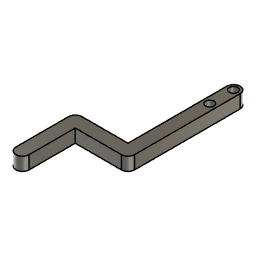
Grabing_Stick2_ver4 v4 (Autodesk Fusion 360 design; units mm, degrees)
Autodesk Fusion 360 part; units mm, degrees
sketch "스케치1" plane through (0, 0, 0) normal (0, 0, 1) x (1, 0, 0)
  line L0 (-2.5, 25) -> (-2.5, -15)
  arc A0 (-2.5, -15) -> (2.5, -15) centre (0, -15) ccw
  line L1 (2.5, -15) -> (2.5, 25)
  arc A1 (2.5, 25) -> (-2.5, 25) centre (0, 25) ccw
  line L2 (0, 25) -> (0, -15) construction
  line L3 (0, -12.5) -> (-20, -12.5)
  arc A2 (-20, -12.5) -> (-20, -17.5) centre (-20, -15) ccw
  line L4 (-20, -17.5) -> (0, -17.5)
  arc A3 (0, -17.5) -> (0, -12.5) centre (0, -15) ccw
  line L5 (0, -15) -> (-20, -15) construction
  line L6 (-22.5, -15) -> (-22.5, -35)
  arc A4 (-22.5, -35) -> (-17.5, -35) centre (-20, -35) ccw
  line L7 (-17.5, -35) -> (-17.5, -15)
  arc A5 (-17.5, -15) -> (-22.5, -15) centre (-20, -15) ccw
  line L8 (-20, -15) -> (-20, -35) construction
  circle A6 centre (0, 25) radius 1.6
  line L9 (-10, 16) -> (11, 16)
  circle A7 centre (0, 16) radius 1.6
  dimension "d1" = 5
  dimension "d2" = 5
  dimension "d3" = 5
  dimension "d4" = 3.2
  dimension "d5" = 9
  dimension "d6" = 3.2
  dimension "d9" = 20
  constraint tangent L0 A0
  constraint tangent A0 L1
  constraint parallel L0 L1
  constraint tangent L1 A1
  constraint tangent L0 A1
  constraint vertical L2
  constraint tangent L3 A2
  constraint tangent A2 L4
  constraint parallel L3 L4
  constraint tangent L4 A3
  constraint tangent L3 A3
  constraint perpendicular L2 L5
  constraint coincident A0.centre L2.end
  constraint tangent L6 A4
  constraint tangent A4 L7
  constraint parallel L6 L7
  constraint tangent L7 A5
  constraint tangent L6 A5
  constraint perpendicular L4 L8
  constraint coincident A2.centre L5.end
  constraint concentric A1 A6
  constraint perpendicular L1 L9
  constraint coincident L9 A7.centre
  constraint coincident L2 A7.centre
  measures "d1" diameter of A0
  measures "d2" diameter of A2
  measures "d3" diameter of A4
  measures "d4" diameter of A6
  measures "d5" distance of A1.centre L9
  measures "d6" diameter of A7
  measures "d9" distance of A0.centre A2.centre
extrude "돌출1" add sketch "스케치1" along normal blind 5 contours L0 L1 A1 L9 A7 | L0 L1 L3 A3 L9 A7 | L0 A0 L3 A3 | L0 A0 L3 L4 L7 A5 | A2 L4 L7 A5 | A2 L4 L6 A4 L7
